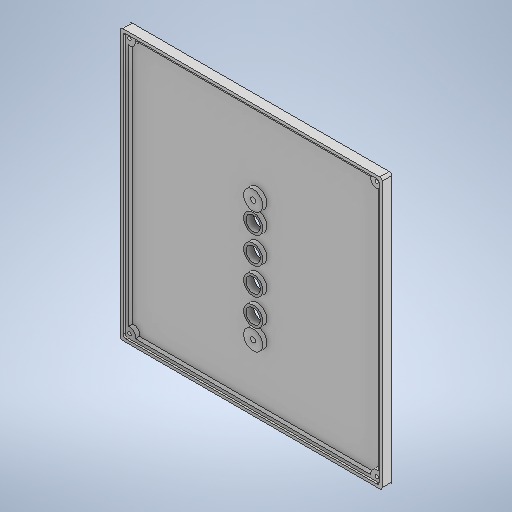
# Autodesk Inventor part: BasePlate
Saved by Autodesk Inventor 2025 (Build 290162000, 162)
## iProperties
Created: 2024-06-17
Part Number: BasePlate
Material: Generic
Document SubType Name: Modeling
Designer: devon
Density: 1 g/cm^3
Appearance: Default
Author: devon
Autodesk Inventor part; units mm, degrees
ref_plane "YZ Plane" through (0, 0, 0) normal (1, 0, 0) x (0, 1, 0)
ref_plane "XZ Plane" through (0, 0, 0) normal (0, 1, 0) x (-1, 0, 0)
ref_plane "XY Plane" through (0, 0, 0) normal (0, 0, 1) x (1, 0, 0)
sketch "Sketch1" plane through (0, 0, 0) normal (0, 0, 1) x (1, 0, 0)
  line L0 (-110, -113.5) -> (110, -113.5)
  line L1 (110, -113.5) -> (110, 113.5)
  line L2 (110, 113.5) -> (-110, 113.5)
  line L3 (-110, 113.5) -> (-110, -113.5)
  line L4 (-110, -113.5) -> (110, 113.5) construction
  line L5 (110, -113.5) -> (-110, 113.5) construction
  point P0 (0, 0)
  dimension "d0" = 220
  dimension "d1" = 227
  constraints: 12 end point, 2 midpoint, 2 parallel, 1 horizontal, 1 perpendicular
  measures "d0" distance of L1.end L2.end
  measures "d1" distance of L0.end L1.end
extrude "Extrusion1" add sketch "Sketch1" along normal blind 8
sketch "Sketch2" plane through (0, 0, 8) normal (0, 0, 1) x (1, 0, 0)
  line L0 (-107.55, -111.05) -> (107.55, -111.05)
  line L1 (107.55, -111.05) -> (107.55, 111.05)
  line L2 (107.55, 111.05) -> (-107.55, 111.05)
  line L3 (-107.55, 111.05) -> (-107.55, -111.05)
  line L4 (-107.55, -111.05) -> (107.55, 111.05) construction
  line L5 (107.55, -111.05) -> (-107.55, 111.05) construction
  point P0 (0, 0)
  dimension "d4" = 215.1
  dimension "d5" = 222.1
  constraints: 12 end point, 2 midpoint, 2 parallel, 1 horizontal, 1 perpendicular
  measures "d4" distance of L1.end L2.end
  measures "d5" distance of L0.end L1.end
extrude "Extrusion2" cut sketch "Sketch2" against normal blind 1.6
sketch "Sketch3" plane through (0, 0, 6.4) normal (0, 0, 1) x (1, 0, 0)
  line L0 (-105, -108.5) -> (105, -108.5)
  line L1 (105, -108.5) -> (105, 108.5)
  line L2 (105, 108.5) -> (-105, 108.5)
  line L3 (-105, 108.5) -> (-105, -108.5)
  line L4 (-105, -108.5) -> (105, 108.5) construction
  line L5 (105, -108.5) -> (-105, 108.5) construction
  point P0 (0, 0)
  dimension "d8" = 210
  dimension "d9" = 217
  constraints: 12 end point, 2 midpoint, 2 parallel, 1 horizontal, 1 perpendicular
  measures "d8" distance of L1.end L2.end
  measures "d9" distance of L0.end L1.end
extrude "Extrusion3" cut sketch "Sketch3" against normal blind 3.5
fillet "Fillet1" radius 2 8 edges at (-107.55, -111.05, 7.2) (-110, -113.5, 4) (110, -113.5, 4) (107.55, -111.05, 7.2) (110, 113.5, 4) (107.55, 111.05, 7.2) (-110, 113.5, 4) (-107.55, 111.05, 7.2)
sketch "Sketch4" plane through (0, 0, 2.9) normal (0, 0, 1) x (1, 0, 0)
  circle A0 centre (-103.9, 107.4) radius 5
  circle A1 centre (-103.9, -107.4) radius 5
  line L0 (-105.55, 111.05) -> (105.55, 111.05) projected
  circle A2 centre (103.9, 107.4) radius 5
  line L1 (107.55, 109.05) -> (107.55, -109.05) projected
  circle A3 centre (103.9, -107.4) radius 5
  line L2 (-107.55, -109.05) -> (-107.55, 109.05) projected
  point P0 (0, 0)
  dimension "d13" = 10
  dimension "d14" = 10
  dimension "d15" = 214.8
  dimension "d16" = 3.65
  dimension "d17" = 10
  dimension "d18" = 207.8
  dimension "d19" = 3.65
  dimension "d20" = 10
  dimension "d21" = 3.65
  dimension "d22" = 214.8
  dimension "d23" = 207.8
  dimension "d24" = 3.65
  constraints: 4 centre point
  measures "d13" diameter of A0
  measures "d14" diameter of A1
  measures "d15" distance of A1.centre A0.centre
  measures "d16" distance from line of L0 A0.centre
  measures "d17" diameter of A2
  measures "d18" distance of A2.centre A0.centre
  measures "d19" distance from line of L1 A2.centre
  measures "d20" diameter of A3
  measures "d21" distance from line of L0 A2.centre
  measures "d22" distance of A3.centre A2.centre
  measures "d23" distance of A3.centre A1.centre
  measures "d24" distance from line of L2 A1.centre
extrude "Extrusion4" add sketch "Sketch4" along normal blind 3.5
sketch "Sketch5" plane through (0, 0, 6.4) normal (0, 0, 1) x (1, 0, 0)
  arc A0 (-105, 102.5225) -> (-99.0225, 108.5) centre (-103.9, 107.4) ccw projected
  circle A1 centre (-103.9, 107.4) radius 1.4
  arc A2 (99.0225, 108.5) -> (105, 102.5225) centre (103.9, 107.4) ccw projected
  circle A3 centre (103.9, 107.4) radius 1.4
  arc A4 (105, -102.5225) -> (99.0225, -108.5) centre (103.9, -107.4) ccw projected
  circle A5 centre (103.9, -107.4) radius 1.4
  arc A6 (-99.0225, -108.5) -> (-105, -102.5225) centre (-103.9, -107.4) ccw projected
  circle A7 centre (-103.9, -107.4) radius 1.4
  point P0 (0, 0)
  dimension "d27" = 2.8
  dimension "d28" = 2.8
  dimension "d29" = 2.8
  dimension "d30" = 2.8
  constraints: 4 centre point, 4 coincident
  measures "d27" diameter of A1
  measures "d28" diameter of A3
  measures "d29" diameter of A5
  measures "d30" diameter of A7
extrude "Extrusion5" cut sketch "Sketch5" against normal blind 3.5
sketch "Sketch6" plane through (0, 0, 2.9) normal (0, 0, 1) x (1, 0, 0)
  circle A0 centre (0, -59.795) radius 8
  line L0 (105.55, -111.05) -> (-105.55, -111.05) projected
  circle A1 centre (0, 41.85) radius 8
  line L1 (-105.55, 111.05) -> (105.55, 111.05) projected
  circle A2 centre (0, -42.5) radius 8
  circle A3 centre (0, -20) radius 8
  circle A4 centre (0, 2.5) radius 8
  circle A5 centre (0, 25) radius 8
  point P0 (0, 0)
  dimension "d33" = 16
  dimension "d34" = 51.255
  dimension "d35" = 16
  dimension "d36" = 69.2
  dimension "d37" = 16
  dimension "d38" = 68.55
  dimension "d39" = 16
  dimension "d40" = 16
  dimension "d41" = 16
  dimension "d42" = 22.5
  dimension "d43" = 22.5
  dimension "d44" = 22.5
  constraints: 6 centre point
  measures "d33" diameter of A0
  measures "d34" distance from line of L0 A0.centre
  measures "d35" diameter of A1
  measures "d36" distance from line of L1 A1.centre
  measures "d37" diameter of A2
  measures "d38" distance from line of L0 A2.centre
  measures "d39" diameter of A3
  measures "d40" diameter of A4
  measures "d41" diameter of A5
  measures "d42" distance of A3.centre A2.centre
  measures "d43" distance of A3.centre A4.centre
  measures "d44" distance of A4.centre A5.centre
extrude "Extrusion6" add sketch "Sketch6" along normal blind 3.5
sketch "Sketch7" plane through (0, 41.85, 6.4) normal (0, 0, 1) x (1, 0, 0)
  circle A0 centre (0, 0) radius 8 projected
  circle A1 centre (0, 0) radius 2.1
  circle A2 centre (0, -16.85) radius 8 projected
  circle A3 centre (0, -16.85) radius 6
  circle A4 centre (0, -39.35) radius 8 projected
  circle A5 centre (0, -39.35) radius 6
  circle A6 centre (0, -61.85) radius 8 projected
  circle A7 centre (0, -61.85) radius 6
  circle A8 centre (0, -84.35) radius 8 projected
  circle A9 centre (0, -84.35) radius 6
  circle A10 centre (0, -101.645) radius 8 projected
  circle A11 centre (0, -101.645) radius 2.1
  point P0 (0, -41.85)
  dimension "d47" = 4.2
  dimension "d48" = 12
  dimension "d49" = 12
  dimension "d50" = 12
  dimension "d51" = 12
  dimension "d52" = 4.2
  constraints: 6 centre point, 6 coincident
  measures "d47" diameter of A1
  measures "d48" diameter of A3
  measures "d49" diameter of A5
  measures "d50" diameter of A7
  measures "d51" diameter of A9
  measures "d52" diameter of A11
extrude "Extrusion7" cut sketch "Sketch7" against normal through all contours A1 | A3 | A5 | A7 | A9 | A11
body "Solid1"
